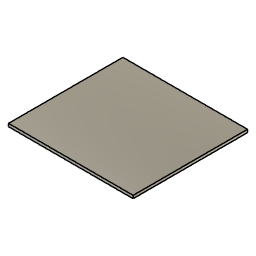
CAD (Autodesk Fusion 360 archive; units mm, degrees)
design "Starter PCB"
description: KiCad electronic assembly
part number: Starter_1 1
Autodesk Fusion 360 part; units mm, degrees
sketch "Sketch1" plane through (0, 0, 1.51) normal (0, 0, 1) x (-1, 0, 0)
  line L0 (-85.24, 172.1) -> (-171.73, 172.1)
  line L1 (-171.73, 172.1) -> (-171.73, 92.74)
  line L2 (-171.73, 92.74) -> (-85.24, 92.74)
  line L3 (-85.24, 92.74) -> (-85.24, 172.1)
  circle A0 centre (-96.139, 143.129) radius 0.85
  circle A1 centre (-101.219, 143.129) radius 2
  circle A2 centre (-97.409, 140.589) radius 0.75
  circle A3 centre (-106.299, 143.129) radius 0.85
  circle A4 centre (-103.759, 138.049) radius 0.75
  circle A5 centre (-153.67, 162.052) radius 0.85
  circle A6 centre (-158.75, 162.052) radius 2
  circle A7 centre (-154.94, 159.512) radius 0.75
  circle A8 centre (-163.83, 162.052) radius 0.85
  circle A9 centre (-161.29, 156.972) radius 0.75
  circle A10 centre (-153.67, 142.875) radius 0.85
  circle A11 centre (-158.75, 142.875) radius 2
  circle A12 centre (-154.94, 140.335) radius 0.75
  circle A13 centre (-163.83, 142.875) radius 0.85
  circle A14 centre (-161.29, 137.795) radius 0.75
  circle A15 centre (-96.139, 123.952) radius 0.85
  circle A16 centre (-97.409, 121.412) radius 0.75
  circle A17 centre (-101.219, 123.952) radius 2
  circle A18 centre (-106.299, 123.952) radius 0.85
  circle A19 centre (-103.759, 118.872) radius 0.75
  circle A20 centre (-115.316, 123.952) radius 0.85
  circle A21 centre (-116.586, 121.412) radius 0.75
  circle A22 centre (-120.396, 123.952) radius 2
  circle A23 centre (-125.476, 123.952) radius 0.85
  circle A24 centre (-122.936, 118.872) radius 0.75
  circle A25 centre (-96.139, 104.775) radius 0.85
  circle A26 centre (-101.219, 104.775) radius 2
  circle A27 centre (-106.299, 104.775) radius 0.85
  circle A28 centre (-97.409, 102.235) radius 0.75
  circle A29 centre (-103.759, 99.695) radius 0.75
  circle A30 centre (-115.316, 104.775) radius 0.85
  circle A31 centre (-120.396, 104.775) radius 2
  circle A32 centre (-125.476, 104.775) radius 0.85
  circle A33 centre (-116.586, 102.235) radius 0.75
  circle A34 centre (-122.936, 99.695) radius 0.75
  circle A35 centre (-134.493, 123.952) radius 0.85
  circle A36 centre (-135.763, 121.412) radius 0.75
  circle A37 centre (-139.573, 123.952) radius 2
  circle A38 centre (-144.653, 123.952) radius 0.85
  circle A39 centre (-142.113, 118.872) radius 0.75
  circle A40 centre (-153.67, 123.952) radius 0.85
  circle A41 centre (-158.75, 123.952) radius 2
  circle A42 centre (-154.94, 121.412) radius 0.75
  circle A43 centre (-163.83, 123.952) radius 0.85
  circle A44 centre (-161.29, 118.872) radius 0.75
  circle A45 centre (-134.493, 104.775) radius 0.85
  circle A46 centre (-139.573, 104.775) radius 2
  circle A47 centre (-144.653, 104.775) radius 0.85
  circle A48 centre (-135.763, 102.235) radius 0.75
  circle A49 centre (-142.113, 99.695) radius 0.75
  circle A50 centre (-152.525, 110.98) radius 0.4445
  circle A51 centre (-152.525, 108.44) radius 0.4445
  circle A52 centre (-152.525, 105.9) radius 0.4445
  circle A53 centre (-167.765, 110.98) radius 0.4445
  circle A54 centre (-167.765, 108.44) radius 0.4445
  circle A55 centre (-167.765, 105.9) radius 0.4445
  circle A56 centre (-152.525, 103.36) radius 0.4445
  circle A57 centre (-152.525, 100.82) radius 0.4445
  circle A58 centre (-152.525, 98.28) radius 0.4445
  circle A59 centre (-152.525, 95.74) radius 0.4445
  circle A60 centre (-167.765, 103.36) radius 0.4445
  circle A61 centre (-167.765, 100.82) radius 0.4445
  circle A62 centre (-167.765, 98.28) radius 0.4445
  circle A63 centre (-167.765, 95.74) radius 0.4445
  line L4 (-85.24, 92.74) -> (-171.73, 92.74)
  line L5 (-171.73, 92.74) -> (-171.73, 172.1)
  line L6 (-171.73, 172.1) -> (-85.24, 172.1)
  line L7 (-85.24, 172.1) -> (-85.24, 92.74)
  constraint horizontal L4
  constraint vertical L5
  constraint horizontal L6
  constraint vertical L7
  constraint coincident L0.end L1.start
  constraint coincident L2.end L3.start
extrude "Extrude1" add sketch "Sketch1" along normal blind 2 contours L0 L1 L2 L3 L4 L5 L6 L7 | A0 | A1 | A2 | A3 | A4 | A5 | A6 | A7 | A8 | A9 | A10 | A11 | A12 | A13 | A14 | A15 | A16 | A17 | A18 | A19 | A20 | A21 | A22 | A23 | A24 | A25 | A26 | A27 | A28 | A29 | A30 | A31 | A32 | A33 | A34 | A35 | A36 | A37 | A38 | A39 | A40 | A41 | A42 | A43 | A44 | A45 | A46 | A47 | A48 | A49 | A50 | A51 | A52 | A53 | A54 | A55 | A56 | A57 | A58 | A59 | A60 | A61 | A62 | A63
